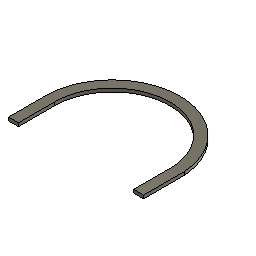
Nose Bridge (Autodesk Fusion 360 design; units mm, degrees)
Autodesk Fusion 360 part; units mm, degrees
sketch "Sketch1" plane through (0, 0, 0) normal (0, 1, 0) x (1, 0, 0)
  line L0 (0, 0) -> (174, 0)
  line L1 (174, 0) -> (174, 102)
  line L2 (174, 102) -> (0, 102)
  line L3 (0, 102) -> (0, 0)
  line L4 (87, 102) -> (87, 0) construction
  arc A0 (26, 54) -> (0, 0) centre (69.0769, 0) ccw
  arc A1 (65, 80) -> (26, 54) centre (197.4493, -160.9239) ccw
  arc A2 (148, 54) -> (109, 80) centre (-23.4493, -160.9239) ccw
  arc A3 (174, 0) -> (148, 54) centre (104.9231, 0) ccw
  arc A4 (109, 80) -> (65, 80) centre (87, 80) ccw
  arc A5 (184, 0) -> (154.2361, 61.8174) centre (104.9231, 0) ccw
  arc A6 (154.2361, 61.8174) -> (118.3954, 86.1912) centre (-23.4493, -160.9239) ccw
  arc A7 (118.3954, 86.1912) -> (55.6046, 86.1912) centre (87, 80) ccw
  arc A8 (55.6046, 86.1912) -> (19.7639, 61.8174) centre (197.4493, -160.9239) ccw
  arc A9 (19.7639, 61.8174) -> (-10, 0) centre (69.0769, 0) ccw
  line L5 (-10, 0) -> (0, 0)
  line L6 (0, 0) -> (0, -30)
  line L7 (0, -30) -> (-10, -30)
  line L8 (-10, -30) -> (-10, 0)
  line L9 (174, 0) -> (184, 0)
  line L10 (184, 0) -> (184, -30)
  line L11 (184, -30) -> (174, -30)
  line L12 (174, -30) -> (174, 0)
  point P0 (26, 54)
  point P1 (65, 80)
  point P2 (148, 54)
  point P3 (109, 80)
  dimension "d1" = 174
  dimension "d2" = 102
  dimension "d3" = 54
  dimension "d5" = 61
  dimension "d6" = 22
  dimension "d7" = 80
  dimension "d8" = 10
  dimension "d9" = 30
  dimension "d10" = 30
  constraint horizontal L0
  constraint vertical L1
  constraint horizontal L2
  constraint vertical L3
  constraint coincident L0.start L3.end
  constraint midpoint L2 L4.start
  constraint midpoint L0 L4.end
  constraint tangent L3 A0
  constraint coincident P0 A0.start
  constraint tangent A0 A1
  constraint coincident P1 A1.start
  constraint symmetric P0 L4 P2
  constraint symmetric L4 P1 P3
  constraint symmetric L4 L0.start L0.end
  constraint symmetric L4 P0 P2
  constraint symmetric L4 A0 A3
  constraint symmetric L4 A1 A2
  constraint coincident L4.start A4
  constraint tangent L2 A4
  constraint coincident P3 A2.end
  constraint horizontal L5
  constraint vertical L6
  constraint horizontal L7
  constraint vertical L8
  constraint horizontal L9
  constraint vertical L10
  constraint horizontal L11
  constraint vertical L12
  constraint coincident A5.start L10
  constraint coincident L0.start L6
  measures "d1" distance of L0.start L0.end
  measures "d2" distance of L0.start L2.end
  measures "d3" distance of L0 P0
  measures "d5" distance of P0 L4
  measures "d6" distance of L4 P1 A5
  measures "d7" distance of L0 P1
  measures "d9" distance of A9.end L7.end
  measures "d10" distance of L0.end L11.end
sketch "Sketch2" plane through (0, 0, 0) normal (0, 1, 0) x (1, 0, 0)
  arc A0 (26, 54) -> (0, 0) centre (69.0769, 0) ccw
  arc A1 (65, 80) -> (26, 54) centre (197.4493, -160.9239) ccw
  arc A2 (109, 80) -> (65, 80) centre (87, 80) ccw
  arc A3 (148, 54) -> (109, 80) centre (-23.4493, -160.9239) ccw
  arc A4 (174, 0) -> (148, 54) centre (104.9231, 0) ccw
  line L0 (174, -30) -> (174, 0)
  line L1 (184, -30) -> (174, -30)
  line L2 (184, 0) -> (184, -30)
  arc A5 (184, 0) -> (154.2361, 61.8174) centre (104.9231, 0) ccw
  arc A6 (154.2361, 61.8174) -> (118.3954, 86.1912) centre (-23.4493, -160.9239) ccw
  arc A7 (118.3954, 86.1912) -> (55.6046, 86.1912) centre (87, 80) ccw
  arc A8 (55.6046, 86.1912) -> (19.7639, 61.8174) centre (197.4493, -160.9239) ccw
  arc A9 (19.7639, 61.8174) -> (-10, 0) centre (69.0769, 0) ccw
  line L3 (-10, -30) -> (-10, 0)
  line L4 (0, -30) -> (-10, -30)
  line L5 (0, 0) -> (0, -30)
sketch "Sketch3" plane through (0, 0, 0) normal (0, 1, 0) x (1, 0, 0)
  arc A0 (118.3954, 86.1912) -> (55.6046, 86.1912) centre (87, 80) ccw
  arc A1 (55.6046, 86.1912) -> (19.7639, 61.8174) centre (197.4493, -160.9239) ccw
  arc A2 (19.7639, 61.8174) -> (-10, 0) centre (69.0769, 0) ccw
  line L0 (-10, -30) -> (-10, 0)
  arc A3 (154.2361, 61.8174) -> (118.3954, 86.1912) centre (-23.4493, -160.9239) ccw
  arc A4 (184, 0) -> (154.2361, 61.8174) centre (104.9231, 0) ccw
  line L1 (184, 0) -> (184, -30)
  line L2 (184, -30) -> (174, -30)
  line L3 (0, -30) -> (-10, -30)
  line L4 (0, 0) -> (0, -30)
  arc A5 (26, 54) -> (0, 0) centre (69.0769, 0) ccw
  arc A6 (65, 80) -> (26, 54) centre (197.4493, -160.9239) ccw
  arc A7 (109, 80) -> (65, 80) centre (87, 80) ccw
  arc A8 (148, 54) -> (109, 80) centre (-23.4493, -160.9239) ccw
  arc A9 (174, 0) -> (148, 54) centre (104.9231, 0) ccw
  line L5 (174, -30) -> (174, 0)
  line L6 (-10, -30) -> (-10, 35.6948)
  line L7 (-10, 35.6948) -> (87, 123.0677)
  line L8 (87, 123.0677) -> (184, 35.6948)
  line L9 (184, 35.6948) -> (184, -30)
  line L10 (-10, -30) -> (0, -30)
  line L11 (0, 24.7023) -> (87, 103.0677)
  line L12 (87, 103.0677) -> (174, 24.7023)
  line L13 (0, 24.7023) -> (0, -30)
  line L14 (174, 24.7023) -> (174, -30)
  line L15 (-10, -30) -> (0, -30)
  line L16 (174, -30) -> (184, -30)
  line L17 (184, -30) -> (189, -30)
  line L18 (189, -30) -> (189, 31.191)
  line L19 (189, 31.191) -> (184, 35.6948)
  line L20 (-10, 35.6948) -> (-15, 31.191)
  line L21 (-15, 31.191) -> (-15, -30)
  line L22 (-15, -30) -> (-10, -30)
  dimension "d11" = 20
  dimension "d14" = 5
  dimension "d15" = 5
  constraint coincident L0.start L3.end
  constraint perpendicular L3 L6
  constraint coincident L1.end L2.start
  constraint parallel L1 L9
  constraint horizontal L6.end L8.end
  constraint tangent A0 L8
  constraint tangent A0 L7
  constraint tangent A3 L8
  constraint coincident L3.start L4.end
  constraint coincident L2.end L5.start
  constraint parallel L9 L14
  constraint parallel L6 L13
  constraint horizontal L11.start L12.end
  constraint parallel L8 L12
  constraint parallel L7 L11
  constraint perpendicular L9 L17
  constraint perpendicular L17 L18
  constraint parallel L8 L19
  constraint collinear L7 L20
  constraint perpendicular L3 L21
  constraint perpendicular L0 L22
  measures "d11" distance of L7.end L11.end
  measures "d14" distance of L1.end L17.end
  measures "d15" distance of L0.start L21.end
extrude "Extrude1" add sketch "Sketch3" along normal blind 5 contours A0 A1 A2 L0 A3 A4 L1 L2 L3 L4 A5 A6 A7 A8 A9 L5 L6 L9 L10 L11 L12 L13 L14 L15 L16 | A0 A3 A4 L8 L9 | A0 L7 L8 | A0 A1 A2 L6 L7 | L1 L9 L17 L18 L19 | L0 L6 L20 L21 L22 | A8 A9 L12 | A5 A6 L11 | A7 L12 | A7 L11 makes body 1
sketch "Sketch4" plane through (0, 0, 0) normal (0, 1, 0) x (-1, 0, 0)
  line L0 (-87, -123.0677) -> (15, -31.191)
  line L1 (15, -31.191) -> (15, 30)
  line L2 (15, 30) -> (0, 30)
  line L3 (0, 30) -> (0, -24.7023)
  line L4 (0, -24.7023) -> (-87, -103.0677)
  line L5 (-87, -103.0677) -> (-174, -24.7023)
  line L6 (-174, -24.7023) -> (-174, 30)
  line L7 (-174, 30) -> (-189, 30)
  line L8 (-189, 30) -> (-189, -31.191)
  line L9 (-189, -31.191) -> (-87, -123.0677)
  line L10 (0, -24.7023) -> (-174, -24.7023)
  arc A0 (-189, -31.191) -> (15, -31.191) centre (-87, -24.7023) ccw
  arc A1 (-174, -24.7023) -> (0, -24.7023) centre (-87, -24.7023) ccw
  line L11 (0, -24.7023) -> (15, -24.7023)
  line L12 (15, -24.7023) -> (15, 30)
  line L13 (15, 30) -> (0, 30)
  line L14 (0, 30) -> (0, -24.7023)
  line L15 (-174, -24.7023) -> (-189, -24.7023)
  line L16 (-189, -24.7023) -> (-189, 30)
  line L17 (-189, 30) -> (-174, 30)
  line L18 (-174, 30) -> (-174, -24.7023)
  line L19 (15, -31.191) -> (15, -24.7023)
  line L20 (-189, -24.7023) -> (-189, -31.191)
  point P0 (-87, -24.7023)
  constraint coincident L3.end L4.start
  constraint coincident L5.end L6.start
  constraint midpoint L10 P0
  constraint coincident L0.end L1.start
  constraint coincident P0 A0.centre
  constraint horizontal L11
  constraint vertical L12
  constraint horizontal L13
  constraint vertical L14
  constraint coincident L1.end L2.start
  constraint horizontal L15
  constraint vertical L16
  constraint horizontal L17
  constraint vertical L18
  constraint coincident L7.end L8.start
  constraint coincident L8.end L9.start
extrude "Extrude2" add sketch "Sketch4" against normal blind 5 separate body contours L0 L9 A1 | L0 L9 A0 A1 | L0 L1 A1 L11 L19 | L8 L9 A1 L15 L20 | L1 L2 L3 L11 L12 L13 L14 | L6 L7 L8 L15 L16 L17 L18 makes body 2
hidden bodies 1
